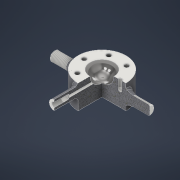
# Autodesk Inventor part: Деталь1
Saved by Autodesk Inventor 2022 (Build 260153000, 153)
## iProperties
Created: 2023-04-26
Part Number: Деталь1
Material: Чугун, литейный
Document SubType Name: Modeling
Designer: lxve_every1
Density: 7.15 g/cm^3
Appearance: Сталь
Author: lxve_every1
Autodesk Inventor part; units mm, degrees
ref_plane "XZ Plane" through (0, 0, 0) normal (0, 1, 0) x (-1, 0, 0)
ref_plane "XY Plane" through (0, 0, 0) normal (0, 0, 1) x (1, 0, 0)
sketch "Эскиз18" plane through (0, 0, 0) normal (0, 0, 1) x (1, 0, 0)
  circle A0 centre (0, 0) radius 50
  dimension "d58" = 100
  constraints: 1 centre point, 1 coincident
  measures "d58" diameter of A0
extrude "Выдавливание4" add sketch "Эскиз18" along normal blind 50
ref_plane "РабПлоскость10" through (0, 0, 25) normal (0, 0, 1) x (1, 0, 0)
sketch "Эскиз19" plane through (0, 0, 25) normal (0, 0, 1) x (1, 0, 0)
  line L0 (0, 0) -> (0, -100)
  line L1 (0, -100) -> (-10, -100)
  line L2 (-10, -100) -> (-10, -65)
  line L3 (-10, -65) -> (-16.5086, -40.7095)
  line L4 (-16.5086, -40.7095) -> (0, -40.7095)
  dimension "d61" = 100
  dimension "d62" = 10
  dimension "d63" = 35
  dimension "d64" = 15
  constraints: 10 end point, 3 perpendicular, 1 point on line, 1 vertical
  measures "d61" distance of L0.start L0.end
  measures "d62" distance of L0.end L1.end
  measures "d63" distance of L1.end L2.end
  measures "d64" angle of L0 L3
revolve "Вращение3" add sketch "Эскиз19" angle 360 about axis through (0, 0, 25) along (0, -1, 0)
thread "Резьба2" size "M20x2.5" class "6g" standard "ISO Metric profile" full length
chamfer "Фаска2" distance 2 angle 45 1 edges at (14.6034, -47.8199, 24.9981)
chamfer "Фаска3" distance 2 angle 45 1 edges at (10, -100, 25)
mirror "Зеркальное отражение2" about plane through (0, 0, 0) normal (0, 1, 0) of "Вращение3", "Фаска2", "Фаска3"
sketch "Эскиз22" plane through (0, 0, 50) normal (0, 0, 1) x (1, 0, 0)
  circle A0 centre (0, 0) radius 25
  line L0 (0, -25) -> (0, 25)
  dimension "d85" = 50
  constraints: 2 end point, 2 point on circle, 1 centre point, 1 coincident, 1 vertical
  measures "d85" diameter of A0
revolve "Вращение4" cut sketch "Эскиз22" angle 360 about axis through (0, -25, 50) along (0, 1, 0) picked at (-8.8525, -4.4917) contours L0 A0
sketch "Эскиз23" plane through (0, 0, 50) normal (0, 0, 1) x (1, 0, 0)
  circle A0 centre (0, 0) radius 37.5
  line L0 (0, 0) -> (32.3421, -18.98)
  dimension "d87" = 75
  constraints: 2 end point, 1 coincident, 3 other
hole "Отверстие4" at (32.3421, -18.98, 50) direction (0, 0, -1) diameter 8.376 depth 20 tip angle 120 countersink diameter 10 countersink angle 120 thread size "M10x1.5" class "6H" standard "ISO Metric profile"
pattern_circular "Круговой массив2" count 6 over 360 about axis through (0, 0, 0) along (0, 0, 1) of "Отверстие4"
ref_plane "РабПлоскость12" through (50, 0, 0) normal (1, 0, 0) x (0, 1, 0)
sketch "Эскиз28" plane through (50, 0, 0) normal (1, 0, 0) x (0, 1, 0)
  line L0 (0, 0) -> (0, 35.3801)
  line L1 (0, 35.3801) -> (0, 0.3801)
  circle A0 centre (0, 35.3801) radius 10
  dimension "d112" = 35
  dimension "d113" = 20
  constraints: 4 end point, 1 centre point, 1 coincident, 1 point on line, 1 vertical
  measures "d112" distance of L0.end L1.end
  measures "d113" diameter of A0
extrude "Выдавливание9" add sketch "Эскиз28" along normal blind 50 and the other way blind 15.25
chamfer "Фаска4" distance 5 angle 45 3 edges at (48.9898, -10, 35.382) (49.4151, 7.6255, 41.8494) (49.4151, 7.6255, 28.9109)
sketch "Эскиз29" plane through (100, 0, 35.3801) normal (1, 0, 0) x (0, 0, -1)
  point P0 (35.3801, 0)
  point P1 (-0.0268, -0.0194)
hole "Отверстие5" at (100, -0.0194, 35.4069) direction (-1, 0, 0) diameter 10.106 depth 30 tip angle 120 countersink diameter 12 countersink angle 90 thread size "M12x1.75" class "6H" standard "ISO Metric profile"
sketch "Эскиз30" plane through (100, 0, 35.3801) normal (1, 0, 0) x (0, 0, -1)
  circle A0 centre (0, 0) radius 2.5
  point P0 (35.3801, 0)
  dimension "d128" = 5
  constraints: 1 centre point
  measures "d128" diameter of A0
extrude "Выдавливание10" cut sketch "Эскиз30" against normal blind 89.25
